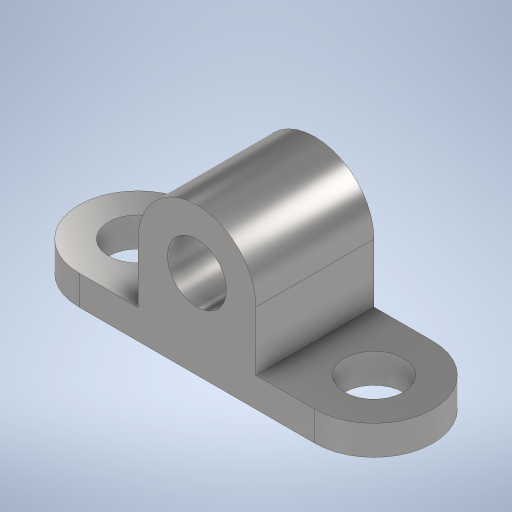
# Autodesk Inventor part: practice2
Saved by Autodesk Inventor 2024 (Build 280153000, 153)
## iProperties
Created: 2024-02-14
Part Number: practice2
Material: Stahl, Guss
Document SubType Name: Modeling
Designer: ffogue
Density: 7.85 g/cm^3
Appearance: Halbpoliert
Author: ffogue
Autodesk Inventor part; units mm, degrees
ref_plane "YZ Plane" through (0, 0, 0) normal (1, 0, 0) x (0, 1, 0)
ref_plane "XZ Plane" through (0, 0, 0) normal (0, 1, 0) x (-1, 0, 0)
ref_plane "XY Plane" through (0, 0, 0) normal (0, 0, 1) x (1, 0, 0)
sketch "Skizze1" plane through (0, 0, 0) normal (0, 0, 1) x (1, 0, 0)
  line L0 (0, 0) -> (80, 0) construction
  line L1 (0, -20) -> (80, -20)
  line L2 (80, 20) -> (0, 20)
  arc A0 (0, 20) -> (0, -20) centre (0, 0) ccw
  arc A1 (80, -20) -> (80, 20) centre (80, 0) ccw
  point P0 (40, 0)
  dimension "d0" = 80
  dimension "d1" = 40
  constraints: 8 end point, 4 point on circle, 4 tangent, 2 centre point, 1 coincident, 1 horizontal, 1 midpoint, 1 parallel
  measures "d0" distance of L0.start L0.end
  measures "d1" distance between parallel lines of L1 L2
extrude "Extrusion1" add sketch "Skizze1" along normal blind 10
sketch "Skizze3" plane through (0, -20, 0) normal (0, -1, 0) x (1, 0, 0)
  line L0 (80, 10) -> (0, 10) projected
  line L1 (20, 10) -> (20, 30)
  arc A0 (60, 30) -> (20, 30) centre (40, 30) ccw
  line L2 (60, 30) -> (60, 10)
  line L3 (80, 0) -> (0, 0) projected
  line L4 (40, 0) -> (40, 30) construction
  dimension "d4" = 20
  dimension "d5" = 20
  constraints: 6 end point, 2 point on circle, 2 point on line, 2 tangent, 2 vertical, 1 centre point, 1 midpoint, 1 parallel
  measures "d4" distance of L2.start L2.end
  measures "d5" radius of A0
extrude "Extrusion2" add sketch "Skizze3" against normal up to surface (40 mm away)
sketch "Skizze4" plane through (0, -20, 0) normal (0, -1, 0) x (1, 0, 0)
  arc A0 (60, 30) -> (20, 30) centre (40, 30) ccw projected
  point P0 (0, 0)
  constraints: 1 coincident
hole "Bohrung1" at (40, -20, 30) direction (0, 1, 0) diameter 20 end through all
sketch "Skizze5" plane through (0, 0, 10) normal (0, 0, 1) x (1, 0, 0)
  arc A0 (0, 20) -> (0, -20) centre (0, 0) ccw projected
  constraints: 1 coincident
hole "Bohrung2" at (0, 0, 10) direction (0, 0, -1) diameter 20 end through all
sketch "Skizze6" plane through (0, 0, 10) normal (0, 0, 1) x (1, 0, 0)
  arc A0 (80, -20) -> (80, 20) centre (80, 0) ccw projected
  point P0 (0, 0)
  point P1 (80, 0)
  constraints: 1 coincident
hole "Bohrung3" at (80, 0, 10) direction (0, 0, -1) diameter 20 end through all
